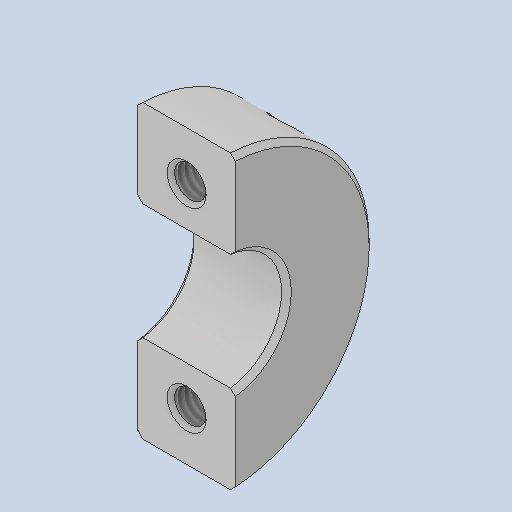
# Autodesk Inventor part: SSCSP12-10p
Saved by Autodesk Inventor 2025.2 (Build 292293000, 293)
## iProperties
Category: PARTsolutions
Company: MISUMI
Created: 2023-12-05
Part Number: SSCSP12-10p
Material: Generic
Catalog Web Link: www.cadenas.de
Description: SCSP,SCSPT,SCSPK,PSCSP,PSCSPT,PSCSPK,SSCSP,SCNPA,SCNPAW,SSCSPT,SSCSPK_p-Set Collars - Separate - Standard, 2 Taps (Coarse Thread), 2 Drill Hole Type
Vendor: MISUMI
Document SubType Name: Modeling
Designer: psAdmin
Manufacturer: MISUMI
Mass: 2.64518 g
Surface Area: 15.0616 cm^2
Volume: 2.64518 cm^3
Density: 1 g/cm^3
Appearance: PSOLRGB-191-191-191
PSOL_IDENT_0: {$CADENAS_DATA/23d-libs/misumi/metric/03_set_collars/scsp_p.prj},240 {VTYP=3D},{NB=SSCSP12-10p},{LIN
PSOL_IDENT_1: A=SSCSP12-10},{NN=SCSP,SCSPT,SCSPK,PSCSP,PSCSPT,PSCSPK,SSCSP,SCNPA,SCNPAW,SSCSPT,SSCSPK_p},{DATE=18.
PSOL_IDENT_2: 06.2021 05:38:59},{GEOMDATE=08.06.2021 04:29:33},{VERSION=},{LINEID=70},{WBVAR=TS,MAT,ST,BS},{WBNUME
PSOL_IDENT_3: RIC=BS}  {NB=SSCSP12-10p},{LINA=SSCSP12-10},{KT=DUMMY},{PN=SSCSP12-10},{TYPE=SSCSP},{TS=S},{MAT=304}
PSOL_IDENT_4: ,{ST=-},{AC=Hexagon Socket Head Cap Screws 2 Pcs. (SUS) },{D=12},{BS=10},{BALG=8,10,12,15},{B1=8,10,
PSOL_IDENT_5: 12,15},{B2=8,10,12},{D1=30},{M=M4},{THMD=4},{THDMIN=3.242},{ST0= '-','-' },{DD=4.5},{R=3.75},{W=1.5}
PSOL_IDENT_6: ,{X=10.0},{Y=5.0},{M1=M4},{M1A=M4},{P1=22.0},{P11=22},{C=0.5},{L=12},{MATA=  '1045','S45C Equivalent'
PSOL_IDENT_7: ,'304','SUS304 Equivalent','2017','A2017(2017 Aluminum)(EN AW-2017_AlCu4MgSi)'   },{THMD1=4},{TS1= '
PSOL_IDENT_8: S', 'Standard','2H','2-Drill Hole','2T','2 Tapped' },{N=5.5},{N1=5.5},{P22=21.0},{P2=21.0},{COL=0.75
PSOL_IDENT_9: ,0.75,0.75,0.00}
NB: SSCSP12-10p
NN: SCSP,SCSPT,SCSPK,PSCSP,PSCSPT,PSCSPK,SSCSP,SCNPA,SCNPAW,SSCSPT,SSCSPK_p
NT: Set Collars - Separate - Standard, 2 Taps (Coarse Thread), 2 Drill Hole Type
NBSYN: $PN.p
LINA: SSCSP12-10
CATALOG: Misumi
PN: SSCSP12-10
TS: Standard
MAT: SUS304 Equivalent
ST: -
D: 12
BS: 10
D1: 30
W: 1.5
X: 10
Y: 5
N: 5.5
P2: 21
SUPPLIER: MISUMI
ARTICLENO: SSCSP12-10p
BOMINFO: SSCSP12-10
CREATOR: CADENAS GmbH
Title: SSCSP12-10
Author: Cadenas PARTsolutions
Comments: Set Collars - Separate - Standard, 2 Taps (Coarse Thread), 2 Drill Hole Type
Autodesk Inventor part; units mm, degrees
sketch "Sketch_1" plane through (0, 0, 0) normal (0, 0, 1) x (1, 0, 0)
  line L0 (5, 0) -> (-5, 0)
  line L1 (-5, 14.5) -> (-5, 6.5)
  line L2 (-5, 6.5) -> (-4.5, 6)
  line L3 (-4.5, 6) -> (4.5, 6)
  line L4 (4.5, 6) -> (5, 6.5)
  line L5 (5, 6.5) -> (5, 14.5)
  line L6 (5, 14.5) -> (4.5, 15)
  line L7 (4.5, 15) -> (-4.5, 15)
  line L8 (-4.5, 15) -> (-5, 14.5)
  constraints: 18 end point
revolve "Revolution1" add sketch "Sketch_1" angle 180 about axis through (5, 0, 0) along (-1, 0, 0)
sketch "Sketch_2" plane through (0, 0, 0) normal (1, 0, 0) x (0, 1, 0)
  line L0 (-16, 0.75) -> (-16, -0.75)
  line L1 (-16, -0.75) -> (16, -0.75)
  line L2 (16, -0.75) -> (16, 0.75)
  line L3 (16, 0.75) -> (-16, 0.75)
  constraints: 8 end point
extrude "Extrusion1" cut sketch "Sketch_2" along normal mid plane 10
sketch "Sketch3" plane through (-4.5, -5.9529, -0.75) normal (0, 0, 1) x (1, 0, 0)
  point P0 (4.5, -4.0471)
hole "Hole1" at (0, -10, -0.75) direction (0, 0, -1) diameter 3.242 depth 15 countersink diameter 4 countersink angle 90 thread size "M4x0.7" class "6H" standard "ISO Metric profile"
sketch "Sketch4" plane through (-4.5, 14.9812, -0.75) normal (0, 0, 1) x (1, 0, 0)
  point P0 (4.5, -4.9812)
hole "Hole2" at (0, 10, -0.75) direction (0, 0, -1) diameter 3.242 depth 15 countersink diameter 4 countersink angle 90 thread size "M4x0.7" class "6H" standard "ISO Metric profile"
ref_plane "2_1_XY" through (0, 0, 0) normal (0, 0, 1) x (1, 0, 0)
ref_plane "2_1_YZ" through (0, 0, 0) normal (1, 0, 0) x (0, 1, 0)
ref_plane "2_1_ZX" through (0, 0, 0) normal (0, 1, 0) x (0, 0, 1)
body "Solid1"
